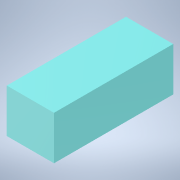
# Autodesk Inventor part: Contenedor A
Saved by Autodesk Inventor 2020.3 (Build 243373000, 373)
## iProperties
Created: 2020-07-23
Part Number: Contenedor A
Material: ABS Plastic
Document SubType Name: Modeling
Designer: juanp
Density: 1.06 g/cm^3
Appearance: Smooth - White
Mass: 364.071 g
Surface Area: 1693.63 cm^2
Volume: 343.463 cm^3
Author: juanp
Autodesk Inventor part; units mm, degrees
ref_plane "YZ Plane" through (0, 0, 0) normal (1, 0, 0) x (0, 1, 0)
ref_plane "XZ Plane" through (0, 0, 0) normal (0, 1, 0) x (-1, 0, 0)
ref_plane "XY Plane" through (0, 0, 0) normal (0, 0, 1) x (1, 0, 0)
sketch "Sketch1" plane through (0, 0, 0) normal (0, 1, 0) x (-1, 0, 0)
  line L0 (0, 0) -> (-80, 0)
  line L1 (-80, 0) -> (-80, -202)
  line L2 (-80, -202) -> (0, -202)
  line L3 (0, -202) -> (0, 0)
  line L4 (-4, -4) -> (-38, -4)
  line L5 (-38, -4) -> (-38, -39.6)
  line L6 (-38, -39.6) -> (-4, -39.6)
  line L7 (-4, -39.6) -> (-4, -4)
  line L8 (-4, -43.6) -> (-38, -43.6)
  line L9 (-38, -43.6) -> (-38, -79.2)
  line L10 (-38, -79.2) -> (-4, -79.2)
  line L11 (-4, -79.2) -> (-4, -43.6)
  line L12 (-4, -83.2) -> (-38, -83.2)
  line L13 (-38, -83.2) -> (-38, -118.8)
  line L14 (-38, -118.8) -> (-4, -118.8)
  line L15 (-4, -118.8) -> (-4, -83.2)
  line L16 (-4, -122.8) -> (-38, -122.8)
  line L17 (-38, -122.8) -> (-38, -158.4)
  line L18 (-38, -158.4) -> (-4, -158.4)
  line L19 (-4, -158.4) -> (-4, -122.8)
  line L20 (-42, -158.4) -> (-42, -122.8)
  line L21 (-42, -122.8) -> (-76, -122.8)
  line L22 (-76, -122.8) -> (-76, -158.4)
  line L23 (-76, -158.4) -> (-42, -158.4)
  line L24 (-76, -118.8) -> (-42, -118.8)
  line L25 (-76, -83.2) -> (-76, -118.8)
  line L26 (-42, -118.8) -> (-42, -83.2)
  line L27 (-42, -83.2) -> (-76, -83.2)
  line L28 (-76, -79.2) -> (-42, -79.2)
  line L29 (-76, -43.6) -> (-76, -79.2)
  line L30 (-42, -79.2) -> (-42, -43.6)
  line L31 (-42, -43.6) -> (-76, -43.6)
  line L32 (-76, -39.6) -> (-42, -39.6)
  line L33 (-42, -4) -> (-76, -4)
  line L34 (-42, -39.6) -> (-42, -4)
  line L35 (-76, -4) -> (-76, -39.6)
  line L36 (-4, -162.4) -> (-76, -162.4)
  line L37 (-76, -162.4) -> (-76, -198)
  line L38 (-76, -198) -> (-4, -198)
  line L39 (-4, -198) -> (-4, -162.4)
  point P0 (0, 0)
  dimension "d8" = 34
  dimension "d9" = 35.6
  dimension "d10" = 4
  dimension "d11" = 4
  dimension "d12" = 39.6
  dimension "d20" = 38
  dimension "d25" = 35.6
  dimension "d26" = 4
  dimension "d27" = 4
  dimension "d28" = 4
  dimension "d29" = 4
  dimension "d30" = 4
  constraints: 80 end point, 6 parallel, 4 horizontal, 3 perpendicular, 2 point on line, 1 vertical, 56 other
  measures "d8" distance of L6.end L6.start
  measures "d9" distance of L6.start L5.start
  measures "d10" distance between parallel lines of L0 L4
  measures "d11" distance between parallel lines of L3 L7
  measures "d12" distance of L4.start L8.start
  measures "d20" distance of L19.start L20.start
  measures "d25" distance of L38.end L36.start
  measures "d26" distance between parallel lines of L18 L36
  measures "d27" distance between parallel lines of L3 L39
  measures "d28" distance between parallel lines of L1 L35
  measures "d29" distance between parallel lines of L1 L37
  measures "d30" distance between parallel lines of L2 L38
extrude "Extrusion1" add sketch "Sketch1" along normal blind 70
sketch "Sketch2" plane through (0, 70, 0) normal (0, 1, 0) x (1, 0, 0)
  line L0 (0, 202) -> (0, 0) projected
  line L1 (0, 0) -> (80, 0) projected
  line L2 (80, 0) -> (80, 202) projected
  line L3 (80, 202) -> (0, 202) projected
extrude "Extrusion2" add sketch "Sketch2" along normal blind 4
fillet "Fillet1" radius 15 36 edges at (76, 70, -180.2) (40, 70, -162.4) (4, 70, -180.2) (40, 70, -198) (76, 70, -21.8) (59, 70, -4) (21, 70, -4) (38, 70, -21.8) (59, 70, -43.6) (76, 70, -61.4) (21, 70, -43.6) (38, 70, -61.4) (21, 70, -83.2) (38, 70, -101) (59, 70, -83.2) (76, 70, -101) (59, 70, -122.8) (76, 70, -140.6) (21, 70, -122.8) (38, 70, -140.6) (4, 70, -21.8) (21, 70, -39.6) (42, 70, -21.8) (59, 70, -39.6) (42, 70, -61.4) (59, 70, -79.2) (4, 70, -61.4) (21, 70, -79.2) (4, 70, -101) (21, 70, -118.8) (42, 70, -101) (59, 70, -118.8) (42, 70, -140.6) (59, 70, -158.4) (4, 70, -140.6) (21, 70, -158.4)
body "Solid1"
